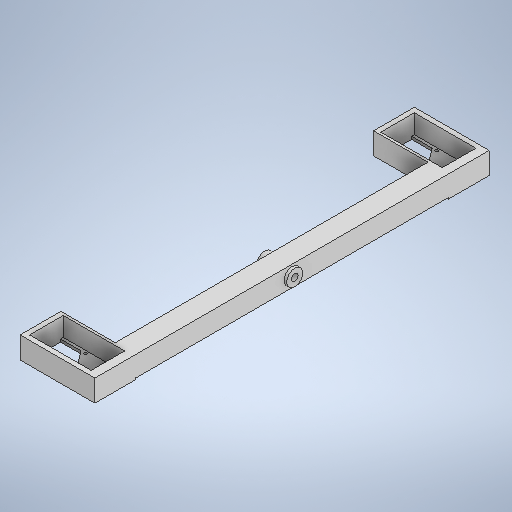
# Autodesk Inventor part: handler
Saved by Autodesk Inventor 2025.3 (Build 293356000, 356)
## iProperties
Created: 2026-03-20
Part Number: handler
Material: Generic
Document SubType Name: Modeling
Designer: ksawe
Density: 1 g/cm^3
Appearance: Default
Author: ksawe
Autodesk Inventor part; units mm, degrees
ref_plane "YZ Plane" through (0, 0, 0) normal (1, 0, 0) x (0, 1, 0)
ref_plane "XZ Plane" through (0, 0, 0) normal (0, 1, 0) x (-1, 0, 0)
ref_plane "XY Plane" through (0, 0, 0) normal (0, 0, 1) x (1, 0, 0)
sketch "Sketch1" plane through (0, 0, 0) normal (0, 1, 0) x (-1, 0, 0)
  line L0 (29.6983, -17.5) -> (-25.3017, -17.5)
  line L1 (-25.3017, -17.5) -> (-25.3017, 12.5)
  line L2 (-25.3017, 12.5) -> (29.6983, 12.5)
  line L3 (29.6983, 12.5) -> (29.6983, -17.5)
  line L4 (29.6983, -17.5) -> (-25.3017, 12.5) construction
  line L5 (-25.3017, -17.5) -> (29.6983, 12.5) construction
  line L6 (26.1983, -15.72) -> (-19.0217, -15.72)
  line L7 (-19.0217, -15.72) -> (-19.0217, 9)
  line L8 (-19.0217, 9) -> (26.1983, 9)
  line L9 (26.1983, 9) -> (26.1983, -15.72)
  line L10 (26.1983, -3.36) -> (-19.0217, -3.36) construction
  circle A0 centre (-16.6614, 6.89) radius 1
  circle A1 centre (7.7883, 7) radius 1
  circle A2 centre (-16.6614, -13.61) radius 1
  circle A3 centre (7.7883, -13.72) radius 1
  circle A4 centre (16.0883, -3.36) radius 9.6 construction
  line L11 (26.1983, 7) -> (11.1983, 7)
  line L12 (11.1983, 7) -> (3.3453, -3.36)
  circle A5 centre (16.0883, -3.36) radius 9.6 construction
  line L13 (26.1983, -13.72) -> (11.1983, -13.72)
  line L14 (11.1983, -13.72) -> (3.3453, -3.36)
  point P0 (2.1983, -2.5)
  dimension "d19" = 55
  dimension "d20" = 30
  dimension "d21" = 45.22
  dimension "d22" = 24.72
  dimension "d23" = 2
  dimension "d24" = 24.45
  dimension "d25" = 18.41
  dimension "d26" = 20.5
  dimension "d27" = 19.2
  dimension "d28" = 10.11
  dimension "d29" = 13
  dimension "d30" = 15
  dimension "d31" = 3.5
  constraints: 30 end point, 6 centre point, 4 midpoint, 4 parallel, 4 symmetric about line, 3 horizontal, 3 point on line, 2 perpendicular, 1 equal radius, 3 other
  measures "d19" distance of L1.end L2.end
  measures "d20" distance of L0.end L1.end
  measures "d21" distance of L7.end L8.end
  measures "d22" distance of L6.end L7.end
  measures "d23" diameter of A1
  measures "d24" distance of A0.centre A1.centre
  measures "d25" distance from line of L9 A1.centre
  measures "d26" distance of A0.centre A2.centre
  measures "d27" diameter of A4
  measures "d28" distance from line of L9 A4.centre
  measures "d29" distance of L11.end L12.end
  measures "d30" distance of L11.start L11.end
  measures "d31" distance between parallel lines of L3 L9
extrude "Extrusion1" add sketch "Sketch1" along normal mid plane 2 contours L0 L1 L2 L3 | L6 L7 L8 L9 L11 L12 L14 L13
extrude "Extrusion2" add sketch "Sketch1" along normal blind 15 contours L0 L1 L2 L3
sketch "Sketch2" plane through (0, 0, 0) normal (0, 1, 0) x (-1, 0, 0)
  line L0 (29.6983, -17.5) -> (-25.3017, -17.5) projected
  line L1 (-25.3017, -17.5) -> (-25.3017, -247.5)
  line L2 (-10.3017, -17.5) -> (-10.3017, -247.5)
  line L3 (-25.3017, -247.5) -> (-10.3017, -247.5)
  point P0 (0, 0)
  dimension "d39" = 230
  dimension "d41" = 15
  constraints: 6 end point, 2 vertical, 1 horizontal, 1 parallel, 1 point on line
  measures "d39" distance of L0.end L1.end
  measures "d41" distance between parallel lines of L2 L1
extrude "Extrusion3" add sketch "Sketch2" along normal blind 2
ref_plane "Work Plane1" through (25.3017, -1, -132.5) normal (0, 0, -1) x (-1, 0, 0)
mirror "Mirror1" about plane through (25.3017, -1, -132.5) normal (0, 0, -1) of "Extrusion1", "Extrusion2"
sketch "Sketch3" plane through (0, 2, 0) normal (0, 1, 0) x (1, 0, 0)
  line L0 (-29.6983, 247.5) -> (25.3017, 247.5) projected
  line L1 (23.3017, 247.5) -> (23.3017, 17.5)
  line L2 (25.3017, 17.5) -> (25.3017, 247.5) projected
  line L3 (12.3017, 247.5) -> (12.3017, 17.5)
  line L4 (10.3017, 247.5) -> (10.3017, 17.5) projected
  line L5 (25.3017, 17.5) -> (25.3017, 247.5) projected
  line L6 (25.3017, 247.5) -> (-29.6983, 247.5) projected
  line L7 (25.3017, 17.5) -> (10.3017, 17.5) projected
  point P0 (0, 0)
  point P1 (10.3017, 167.5)
  dimension "d45" = 2
  dimension "d46" = 2
  constraints: 4 end point, 3 parallel, 2 point on line, 1 perpendicular
  measures "d45" distance between parallel lines of L2 L1
  measures "d46" distance between parallel lines of L4 L3
extrude "Extrusion4" add sketch "Sketch3" along normal blind 13
sketch "Sketch4" plane through (10.3017, 0, -17.5) normal (-1, 0, 0) x (0, 0, 1)
  circle A0 centre (-115, 7.5) radius 2.5
  line L0 (-230, 0) -> (0, 0) projected
  line L1 (-230, 0) -> (-230, 15) projected
  circle A1 centre (-115, 7.5) radius 6
  point P0 (17.5, 0)
  dimension "d49" = 5
  dimension "d50" = 7.5
  dimension "d52" = 12
  dimension "d61" = 115
  constraints: 2 centre point, 1 coincident
  measures "d49" diameter of A0
  measures "d50" distance from line of L0 A0.centre
  measures "d52" diameter of A1
  measures "d61" distance from line of L1 A0.centre
extrude "Extrusion5" add sketch "Sketch4" along normal blind 5 and the other way blind 17 contours A0 | A1
extrude "Extrusion6" cut sketch "Sketch4" along normal blind 5 and the other way blind 17 contours A0
body "Solid1"
